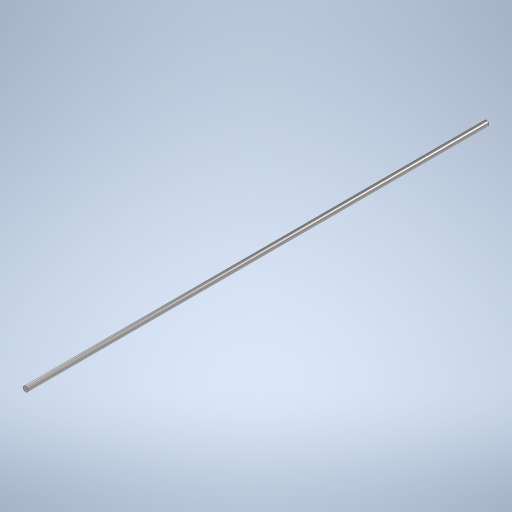
# Autodesk Inventor part: lead screw 8mm 700mm
Saved by Autodesk Inventor 2023.2 (Build 272271000, 271)
## iProperties
Created: 2023-03-29
Part Number: lead screw 8mm 700mm
Material: Stainless Steel
Document SubType Name: Modeling
Designer: dmargari
Density: 8 g/cm^3
Appearance: Semi-Polished
Author: dmargari
Autodesk Inventor part; units mm, degrees
ref_plane "YZ Plane" through (0, 0, 0) normal (1, 0, 0) x (0, 1, 0)
ref_plane "XZ Plane" through (0, 0, 0) normal (0, 1, 0) x (-1, 0, 0)
ref_plane "XY Plane" through (0, 0, 0) normal (0, 0, 1) x (1, 0, 0)
sketch "Sketch1" plane through (0, 0, 0) normal (0, 0, 1) x (1, 0, 0)
  circle A0 centre (6.1326, 8.4757) radius 4
  point P0 (0, 0)
  dimension "d0" = 8
  dimension "d0" = 8
  constraints: 1 centre point
  measures "d0" diameter of A0
extrude "Extrusion1" add sketch "Sketch1" along normal mid plane 700
body "Solid1"
